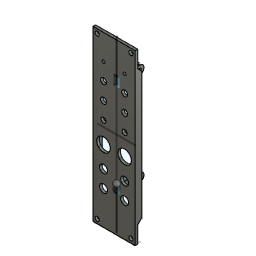
LMNC-DualADSR (Autodesk Fusion 360 design; units mm, degrees)
Autodesk Fusion 360 part; units mm, degrees
note: some values were not read from the file. Set by a fixed rule: which sketch regions a step uses.
sketch "Sketch1" plane through (0, 0, 0) normal (0, 0, 1) x (1, 0, 0)
  line L0 (5, 5) -> (55, 5)
  line L1 (55, 5) -> (55, 205)
  line L2 (55, 205) -> (5, 205)
  line L3 (5, 205) -> (5, 5)
  line L4 (5, 205) -> (5, 200)
  line L5 (5, 200) -> (10, 200)
  circle A0 centre (10, 200) radius 2.5
  line L6 (5, 5) -> (5, 10)
  line L7 (5, 10) -> (10, 10)
  circle A1 centre (10, 10) radius 2.5
  line L8 (30, 205) -> (30, 5)
  circle A2 centre (50, 200) radius 2.5
  circle A3 centre (50, 10) radius 2.5
  dimension "d1" = 50
  dimension "d2" = 200
  dimension "d3" = 5
  dimension "d4" = 5
  constraint horizontal L0
  constraint vertical L1
  constraint horizontal L2
  constraint vertical L3
  constraint coincident L3 L4.end
  constraint perpendicular L3 L5
  constraint coincident L5.end A0.centre
  constraint coincident L3 L6.end
  constraint perpendicular L6 L7
  constraint coincident L7.end A1.centre
  constraint midpoint L2 L8.start
  constraint midpoint L0 L8.end
  constraint symmetric A0 L8 A2
  constraint symmetric A1 L8 A3
  measures "d1" distance of L0.start L0.end
  measures "d2" distance of L0.start L2.end
  measures "d3" diameter of A0
  measures "d4" diameter of A1
extrude "Extrude1" add sketch "Sketch1" along normal blind 3
sketch "Sketch2" plane through (0, 0, 3) normal (0, 0, 1) x (1, 0, 0)
  circle A0 centre (10, 200) radius 2.5
  circle A1 centre (50, 200) radius 2.5
  circle A2 centre (10, 10) radius 2.5
  circle A3 centre (50, 10) radius 2.5
  line L0 (55, 5) -> (55, 205)
  line L1 (55, 205) -> (5, 205)
  line L2 (5, 205) -> (5, 5)
  line L3 (5, 5) -> (55, 5)
  line L4 (5, 205) -> (17.5, 205)
  line L5 (17.5, 205) -> (17.5, 5)
  line L6 (55, 205) -> (42.5, 205)
  line L7 (42.5, 205) -> (42.5, 5)
  line L8 (30, 205) -> (30, 5)
  line L9 (5, 205) -> (5, 185)
  line L10 (5, 5) -> (5, 25)
  line L11 (5, 25) -> (55, 25)
  line L12 (5, 185) -> (55, 185)
  line L13 (17.5, 185) -> (17.5, 175)
  circle A4 centre (17.5, 175) radius 1.75
  line L14 (17.5, 25) -> (17.5, 45)
  circle A5 centre (17.5, 45) radius 4.75
  line L15 (17.5, 45) -> (17.5, 65)
  circle A6 centre (17.5, 65) radius 4.75
  line L16 (17.5, 175) -> (17.5, 155)
  circle A7 centre (17.5, 155) radius 3.5
  line L17 (17.5, 155) -> (17.5, 135)
  circle A8 centre (17.5, 135) radius 3.5
  line L18 (17.5, 135) -> (17.5, 115)
  circle A9 centre (17.5, 115) radius 3
  line L19 (17.5, 115) -> (17.5, 90)
  circle A10 centre (17.5, 90) radius 8
  circle A11 centre (42.5, 175) radius 1.75
  circle A12 centre (42.5, 155) radius 3.5
  circle A13 centre (42.5, 135) radius 3.5
  circle A14 centre (42.5, 115) radius 3
  circle A15 centre (42.5, 90) radius 8
  circle A16 centre (42.5, 65) radius 4.75
  circle A17 centre (42.5, 45) radius 4.75
  dimension "d7" = 12.5
  dimension "d8" = 200
  dimension "d9" = 12.5
  dimension "d10" = 20
  dimension "d11" = 20
  dimension "d12" = 10
  dimension "d13" = 3.5
  dimension "d14" = 20
  dimension "d15" = 9.5
  dimension "d16" = 20
  dimension "d17" = 9.5
  dimension "d18" = 20
  dimension "d19" = 7
  dimension "d20" = 20
  dimension "d21" = 7
  dimension "d22" = 20
  dimension "d23" = 6
  dimension "d24" = 25
  dimension "d25" = 16
  constraint coincident L1.end L2.start
  constraint perpendicular L2 L4
  constraint perpendicular L3 L5
  constraint coincident L0.end L1.start
  constraint perpendicular L0 L6
  constraint coincident L3 L7.end
  constraint perpendicular L3 L7
  constraint midpoint L1 L8.start
  constraint midpoint L3 L8.end
  constraint perpendicular L4 L9
  constraint coincident L2.end L3.start
  constraint perpendicular L3 L10
  constraint coincident L0 L11.end
  constraint perpendicular L0 L11
  constraint coincident L0 L12.end
  constraint perpendicular L0 L12
  constraint coincident L12 L13.start
  constraint coincident L5 L13.start
  constraint perpendicular L12 L13
  constraint coincident L13.end A4.centre
  constraint coincident L5 L14.start
  constraint coincident L11 L14.start
  constraint perpendicular L11 L14
  constraint coincident L14.end A5.centre
  constraint parallel L5 L15
  constraint coincident L15.end A6.centre
  constraint parallel L5 L16
  constraint coincident L16.end A7.centre
  constraint parallel L5 L17
  constraint coincident L17.end A8.centre
  constraint parallel L5 L18
  constraint coincident L18.end A9.centre
  constraint parallel L5 L19
  constraint coincident L19.end A10.centre
  constraint symmetric L8 A4 A11
  constraint symmetric L8 A5 A17
  constraint symmetric L8 A6 A16
  constraint symmetric L8 A7 A12
  constraint symmetric L8 A8 A13
  constraint symmetric L8 A9 A14
  constraint symmetric L8 A10 A15
  measures "d7" distance of L1.end L4.end
  measures "d8" distance of L4.end L5.end
  measures "d9" distance of L0.end L6.end
  measures "d10" distance of L1.end L9.end
  measures "d11" distance of L2.end L10.end
  measures "d12" distance of L13.start L13.end
  measures "d13" diameter of A4
  measures "d14" distance of L14.start L14.end
  measures "d15" diameter of A5
  measures "d16" distance of L14.end L15.end
  measures "d17" diameter of A6
  measures "d18" distance of L13.end L16.end
  measures "d19" diameter of A7
  measures "d20" distance of L16.end L17.end
  measures "d21" diameter of A8
  measures "d22" distance of L17.end L18.end
  measures "d23" diameter of A9
  measures "d24" distance of L18.end L19.end
  measures "d25" diameter of A10
extrude "Extrude2" cut sketch "Sketch2" against normal blind 3 contours L7 A17 | L7 A17 | L7 A11 | L7 A11 | L7 A16 | L7 A16 | L5 L14 A5 L15 | L5 L14 A5 L15 | L7 A12 | L7 A12 | L5 L13 A4 L16 | L5 L13 A4 L16 | L7 A15 | L7 A15 | L5 L15 A6 | L5 L15 A6 | L7 A13 | L7 A13 | L5 L16 A7 L17 | L5 L16 A7 L17 | L7 A14 | L7 A14 | L5 L19 A10 | L5 L19 A10 | L5 L17 A8 L18 | L5 L17 A8 L18 | L5 L18 A9 L19 | L5 L18 A9 L19
sketch "Sketch3" plane through (0, 0, 0) normal (0, 0, -1) x (-1, 0, 0)
  circle A0 centre (-42.5, 135) radius 3.5
  circle A1 centre (-42.5, 45) radius 4.75
  circle A2 centre (-17.5, 115) radius 3
  circle A3 centre (-17.5, 155) radius 3.5
  circle A4 centre (-17.5, 90) radius 8
  circle A5 centre (-42.5, 65) radius 4.75
  circle A6 centre (-42.5, 155) radius 3.5
  circle A7 centre (-42.5, 115) radius 3
  circle A8 centre (-17.5, 45) radius 4.75
  circle A9 centre (-17.5, 135) radius 3.5
  circle A10 centre (-17.5, 175) radius 1.75
  circle A11 centre (-17.5, 65) radius 4.75
  circle A12 centre (-42.5, 90) radius 8
  circle A13 centre (-42.5, 175) radius 1.75
  circle A14 centre (-10, 200) radius 2.5
  circle A15 centre (-50, 200) radius 2.5
  circle A16 centre (-10, 10) radius 2.5
  circle A17 centre (-50, 10) radius 2.5
  line L0 (-55, 205) -> (-55, 5)
  line L1 (-55, 5) -> (-5, 5)
  line L2 (-5, 5) -> (-5, 205)
  line L3 (-5, 205) -> (-55, 205)
  line L4 (-55, 205) -> (-55, 185)
  line L5 (-55, 185) -> (-52, 185)
  line L6 (-52, 185) -> (-52, 25)
  line L7 (-52, 25) -> (-55, 25)
  line L8 (-55, 25) -> (-55, 185)
  line L9 (-30, 205) -> (-30, 5)
  line L10 (-5, 25) -> (-5, 185)
  line L11 (-8, 185) -> (-8, 25)
  line L12 (-8, 25) -> (-5, 25)
  line L13 (-5, 185) -> (-8, 185)
  dimension "d28" = 20
  dimension "d29" = 3
  dimension "d30" = 160
  constraint coincident L0.start L3.end
  constraint perpendicular L3 L4
  constraint horizontal L5
  constraint vertical L6
  constraint horizontal L7
  constraint vertical L8
  constraint midpoint L3 L9.start
  constraint midpoint L1 L9.end
  constraint symmetric L4.end L9 L10.end
  constraint symmetric L5.end L9 L11.start
  constraint symmetric L6.end L9 L11.end
  constraint symmetric L7.end L9 L10.start
  measures "d28" distance of L0.start L4.end
  measures "d29" distance of L4.end L5.end
  measures "d30" distance of L4.end L7.end
extrude "Extrude3" add sketch "Sketch3" along normal blind 5 contours L0 L5 L6 L7 L8 | L2 L10 L11 L12 L13
chamfer "Chamfer1" distance 5 angle 45 4 edges at (6.5, 25, -5) (53.5, 25, -5) (6.5, 185, -5) (53.5, 185, -5)
sketch "Sketch4" plane through (0, 0, 0) normal (1, 0, 0) x (0, 0, -1)
sketch "Sketch5" plane through (0, 0, 0) normal (0, 0, -1) x (-1, 0, 0)
  circle A0 centre (-42.5, 135) radius 3.5
  circle A1 centre (-42.5, 45) radius 4.75
  circle A2 centre (-17.5, 115) radius 3
  circle A3 centre (-17.5, 155) radius 3.5
  circle A4 centre (-17.5, 90) radius 8
  circle A5 centre (-42.5, 65) radius 4.75
  circle A6 centre (-42.5, 155) radius 3.5
  circle A7 centre (-42.5, 115) radius 3
  circle A8 centre (-17.5, 45) radius 4.75
  circle A9 centre (-17.5, 135) radius 3.5
  circle A10 centre (-17.5, 175) radius 1.75
  circle A11 centre (-17.5, 65) radius 4.75
  circle A12 centre (-42.5, 90) radius 8
  circle A13 centre (-42.5, 175) radius 1.75
  circle A14 centre (-10, 200) radius 2.5
  circle A15 centre (-50, 200) radius 2.5
  circle A16 centre (-10, 10) radius 2.5
  circle A17 centre (-50, 10) radius 2.5
  line L0 (-5, 25) -> (-8, 25)
  line L1 (-8, 25) -> (-8, 185)
  line L2 (-8, 185) -> (-5, 185)
  line L3 (-5, 185) -> (-5, 205)
  line L4 (-5, 205) -> (-55, 205)
  line L5 (-55, 205) -> (-55, 185)
  line L6 (-55, 185) -> (-52, 185)
  line L7 (-52, 185) -> (-52, 25)
  line L8 (-52, 25) -> (-55, 25)
  line L9 (-55, 25) -> (-55, 5)
  line L10 (-55, 5) -> (-5, 5)
  line L11 (-5, 5) -> (-5, 25)
  line L12 (-30, 205) -> (-30, 5)
  line L13 (-30, 205) -> (-30, 165)
  line L14 (-30, 5) -> (-30, 50)
  line L15 (-30, 165) -> (-27.5, 165)
  line L16 (-27.5, 165) -> (-27.5, 155)
  line L17 (-27.5, 155) -> (-30, 155)
  line L18 (-30, 155) -> (-30, 165)
  line L19 (-30, 165) -> (-32.5, 165)
  line L20 (-32.5, 165) -> (-32.5, 155)
  line L21 (-32.5, 155) -> (-30, 155)
  line L22 (-30, 155) -> (-30, 165)
  line L23 (-52, 105) -> (-8, 105)
  line L24 (-27.5, 55) -> (-30, 55)
  line L25 (-27.5, 45) -> (-27.5, 55)
  line L26 (-30, 45) -> (-27.5, 45)
  line L27 (-30, 45) -> (-32.5, 45)
  line L28 (-32.5, 45) -> (-32.5, 55)
  line L29 (-32.5, 55) -> (-30, 55)
  dimension "d34" = 40
  dimension "d35" = 45
  dimension "d36" = 2.5
  dimension "d37" = 10
  constraint midpoint L4 L12.start
  constraint midpoint L10 L12.end
  constraint perpendicular L4 L13
  constraint perpendicular L10 L14
  constraint horizontal L15
  constraint vertical L16
  constraint horizontal L17
  constraint vertical L18
  constraint horizontal L19
  constraint vertical L20
  constraint horizontal L21
  constraint vertical L22
  constraint midpoint L7 L23.start
  constraint midpoint L1 L23.end
  constraint symmetric L13.end L23 L26.start
  constraint symmetric L15.end L23 L25.start
  constraint symmetric L16.end L23 L24.start
  constraint symmetric L17.end L23 L24.end
  constraint symmetric L19.end L23 L27.end
  constraint symmetric L20.end L23 L28.end
  measures "d34" distance of L12.start L13.end
  measures "d35" distance of L12.end L14.end
  measures "d36" distance of L13.end L15.end
  measures "d37" distance of L13.end L17.end
extrude "Extrude4" add sketch "Sketch5" along normal blind 30 contours L12 L14 L27 L28 L29 | L12 L14 L24 L25 L26
extrude "Extrude5" add sketch "Sketch5" along normal blind 30 contours L12 L18 L19 L20 L21 L22 | L12 L15 L16 L17 L18 L22
fillet "Fillet1" radius 5 4 edges at (30, 155, -30) (30, 165, -30) (30, 55, -30) (30, 45, -30)
sketch "Sketch6" plane through (27.5, 0, 0) normal (-1, 0, 0) x (0, 0, 1)
  arc A0 (-25, 165) -> (-25, 155) centre (-25, 160) ccw
  line L0 (-25, 155) -> (0, 155)
  line L1 (0, 155) -> (0, 165)
  line L2 (0, 165) -> (-25, 165)
  line L3 (-30, 160) -> (-25, 160)
  line L4 (-30, 50) -> (-25, 50)
  circle A1 centre (-25, 50) radius 1.75
  circle A2 centre (-25, 160) radius 1.75
  dimension "d43" = 3.5
  dimension "d44" = 3.5
  constraint midpoint A0 L3.start
  constraint coincident A0.centre L3.end
  constraint horizontal L4
  constraint coincident L4.end A1.centre
  measures "d43" diameter of A1
  measures "d44" diameter of A2
extrude "Extrude6" cut sketch "Sketch6" against normal blind 5 contours A1 | A2
